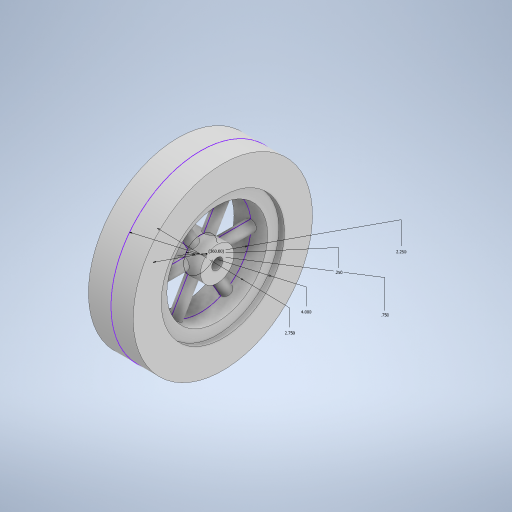
# Autodesk Inventor part: Flywheel
Saved by Autodesk Inventor 2023 (Build 270158000, 158)
## iProperties
Created: 2022-12-28
Part Number: Flywheel
Material: Generic
Document SubType Name: Modeling
Designer: tgr41
Density: 1 g/cm^3
Appearance: Default
Author: tgr41
Autodesk Inventor part; units mm, degrees
ref_plane "YZ Plane" through (0, 0, 0) normal (1, 0, 0) x (0, 1, 0)
ref_plane "XZ Plane" through (0, 0, 0) normal (0, 1, 0) x (-1, 0, 0)
ref_plane "XY Plane" through (0, 0, 0) normal (0, 0, 1) x (1, 0, 0)
sketch "Sketch1" plane through (0, 0, 0) normal (1, 0, 0) x (0, 1, 0)
  circle A0 centre (0, 0) radius 50.8
  circle A1 centre (0, 0) radius 9.525
  circle A2 centre (0, 0) radius 3.175
  circle A3 centre (0, 0) radius 34.925
  circle A4 centre (0, 0) radius 28.575
  line L0 (-3.175, -8.9803) -> (-3.175, -28.3981)
  line L1 (3.175, -8.9803) -> (3.175, -28.3981)
  line L2 (6.1896, -7.2398) -> (23.0059, -16.9487)
  line L3 (9.3646, -1.7405) -> (26.1809, -11.4494)
  line L4 (9.3646, 1.7405) -> (26.1809, 11.4494)
  line L5 (6.1896, 7.2398) -> (23.0059, 16.9487)
  line L6 (3.175, 8.9803) -> (3.175, 28.3981)
  line L7 (-3.175, 8.9803) -> (-3.175, 28.3981)
  line L8 (-6.1896, 7.2398) -> (-23.0059, 16.9487)
  line L9 (-9.3646, 1.7405) -> (-26.1809, 11.4494)
  line L10 (-9.3646, -1.7405) -> (-26.1809, -11.4494)
  line L11 (-6.1896, -7.2398) -> (-23.0059, -16.9487)
  dimension "d31" = 69.85
  dimension "d32" = 101.6
  dimension "d33" = 19.05
  dimension "d34" = 6.35
  dimension "d35" = 57.15
  dimension "d39" = 360
  constraints: 24 end point, 5 centre point, 4 point on circle, 3 coincident, 1 concentric, 1 vertical, 37 other
  measures "d31" diameter of A3
  measures "d32" diameter of A0
  measures "d33" diameter of A1
  measures "d34" diameter of A2
  measures "d35" diameter of A4
extrude "Extrusion7" add sketch "Sketch1" along normal mid plane 25.4 contours A0
extrude "Extrusion8" add sketch "Sketch1" along normal mid plane 19.05 contours A1 | A3
extrude "Extrusion9" add sketch "Sketch1" along normal mid plane 6.35 contours A1 L5 A4 L4 | L3 A4 L2 A1 | A1 L7 A4 L6 | L1 A4 L0 A1 | A1 L9 A4 L8 | L11 A4 L10 A1
fillet "Fillet1" radius 3.175 24 edges at (3.175, 14.5978, -12.0942) (3.175, 17.7728, -6.5949) (-3.175, 14.5978, -12.0942) (3.175, 3.175, -18.6892) (3.175, -3.175, -18.6892) (3.175, -14.5978, -12.0942) (3.175, -17.7728, -6.5949) (3.175, -17.7728, 6.5949) (3.175, -14.5978, 12.0942) (3.175, -3.175, 18.6892) (3.175, 3.175, 18.6892) (3.175, 14.5978, 12.0942) (3.175, 17.7728, 6.5949) (-3.175, -14.5978, 12.0942) (-3.175, -17.7728, 6.5949) (-3.175, -17.7728, -6.5949) (-3.175, -14.5978, -12.0942) (-3.175, -3.175, -18.6892) (-3.175, 3.175, -18.6892) (-3.175, 17.7728, -6.5949) (-3.175, 17.7728, 6.5949) (-3.175, 14.5978, 12.0942) (-3.175, 3.175, 18.6892) (-3.175, -3.175, 18.6892)
body "Solid3"
